Autodesk Fusion 360 part; units mm, degrees
(part 4 of 5)
  line L581 (-46.6267, 18.3537, 609.9137) -> (-48.3447, 10.2533, 610.9671) construction
  line L582 (-48.3447, 10.2533, 610.9671) -> (-50.0626, 2.1529, 612.0205) construction
  line L583 (-50.0626, 2.1529, 612.0205) -> (-49.7012, -6.3796, 613.0739) construction
  line L584 (-49.7012, -6.3796, 613.0739) -> (-47.3042, -14.3056, 614.1273) construction
  line L585 (-47.3042, -14.3056, 614.1273) -> (-44.9073, -22.2315, 615.1807) construction
  line L586 (-44.9073, -22.2315, 615.1807) -> (-40.48, -29.5343, 616.2341) construction
  line L587 (-40.48, -29.5343, 616.2341) -> (-34.5612, -35.325, 617.2875) construction
  line L588 (-34.5612, -35.325, 617.2875) -> (-28.6425, -41.1158, 618.3408) construction
  line L589 (-28.6425, -41.1158, 618.3408) -> (-21.2448, -45.3823, 619.3942) construction
  line L590 (-21.2448, -45.3823, 619.3942) -> (-13.2686, -47.6055, 620.4476) construction
  line L591 (-13.2686, -47.6055, 620.4476) -> (-5.2924, -49.8286, 621.5009) construction
  line L592 (-5.2924, -49.8286, 621.5009) -> (3.2455, -50.0036, 622.5543) construction
  line L593 (3.2455, -50.0036, 622.5543) -> (11.3061, -48.1093, 623.6076) construction
  line L594 (11.3061, -48.1093, 623.6076) -> (19.3665, -46.2151, 624.661) construction
  line L595 (19.3665, -46.2151, 624.661) -> (26.9327, -42.2555, 625.7143) construction
  line L596 (26.9327, -42.2555, 625.7143) -> (33.0837, -36.7125, 626.7677) construction
  line L597 (33.0837, -36.7125, 626.7677) -> (39.2345, -31.1696, 627.821) construction
  line L598 (39.2345, -31.1696, 627.821) -> (43.9574, -24.055, 628.8743) construction
  line L599 (43.9574, -24.055, 628.8743) -> (46.6773, -16.2346, 629.9277) construction
  line L600 (46.6773, -16.2346, 629.9277) -> (49.3973, -8.4143, 630.981) construction
  line L601 (49.3973, -8.4143, 630.981) -> (50.1087, 0.0954, 632.0343) construction
  line L602 (50.1087, 0.0954, 632.0343) -> (48.725, 8.2588, 633.0876) construction
  line L603 (48.725, 8.2588, 633.0876) -> (47.3414, 16.422, 634.1409) construction
  line L604 (47.3414, 16.422, 634.1409) -> (43.8656, 24.2219, 635.1942) construction
  line L605 (43.8656, 24.2219, 635.1942) -> (38.7207, 30.709, 636.2475) construction
  line L606 (38.7207, 30.709, 636.2475) -> (33.5759, 37.1961, 637.3008) construction
  line L607 (33.5759, 37.1961, 637.3008) -> (26.7728, 42.3569, 638.354) construction
  line L608 (26.7728, 42.3569, 638.354) -> (19.1393, 45.5634, 639.4073) construction
  line L609 (19.1393, 45.5634, 639.4073) -> (11.506, 48.7699, 640.4606) construction
  line L610 (11.506, 48.7699, 640.4606) -> (3.0583, 50.0153, 641.5139) construction
  line L611 (3.0583, 50.0153, 641.5139) -> (-5.1756, 49.1482, 642.5671) construction
  line L612 (-5.1756, 49.1482, 642.5671) -> (-13.4094, 48.2812, 643.6204) construction
  line L613 (-13.4094, 48.2812, 643.6204) -> (-21.4122, 45.3034, 644.6736) construction
  line L614 (-21.4122, 45.3034, 644.6736) -> (-28.2102, 40.5774, 645.7269) construction
  line L615 (-28.2102, 40.5774, 645.7269) -> (-35.008, 35.8514, 646.7801) construction
  line L616 (-35.008, 35.8514, 646.7801) -> (-40.5867, 29.3871, 647.8334) construction
  line L617 (-40.5867, 29.3871, 647.8334) -> (-44.2675, 21.971, 648.8866) construction
  line L618 (-44.2675, 21.971, 648.8866) -> (-47.9482, 14.5551, 649.9398) construction
  line L619 (-47.9482, 14.5551, 649.9398) -> (-49.7233, 6.203, 650.993) construction
  line L620 (-49.7233, 6.203, 650.993) -> (-49.3767, -2.0688, 652.0463) construction
  line L621 (-49.3767, -2.0688, 652.0463) -> (-49.0301, -10.3405, 653.0995) construction
  line L622 (-49.0301, -10.3405, 653.0995) -> (-46.5627, -18.5147, 654.1527) construction
  line L623 (-46.5627, -18.5147, 654.1527) -> (-42.2746, -25.5967, 655.2059) construction
  line L624 (-42.2746, -25.5967, 655.2059) -> (-37.9867, -32.6786, 656.2591) construction
  line L625 (-37.9867, -32.6786, 656.2591) -> (-31.8871, -38.6534, 657.3123) construction
  line L626 (-31.8871, -38.6534, 657.3123) -> (-24.7182, -42.7942, 658.3655) construction
  line L627 (-24.7182, -42.7942, 658.3655) -> (-17.5494, -46.935, 659.4186) construction
  line L628 (-17.5494, -46.935, 659.4186) -> (-9.3262, -49.2331, 660.4718) construction
  line L629 (-9.3262, -49.2331, 660.4718) -> (-1.0493, -49.4089, 661.525) construction
  line L630 (-1.0493, -49.4089, 661.525) -> (7.2275, -49.5846, 662.5782) construction
  line L631 (7.2275, -49.5846, 662.5782) -> (15.5406, -47.6378, 663.6313) construction
  line L632 (15.5406, -47.6378, 663.6313) -> (22.8787, -43.8053, 664.6845) construction
  line L633 (22.8787, -43.8053, 664.6845) -> (30.2167, -39.9728, 665.7376) construction
  line L634 (30.2167, -39.9728, 665.7376) -> (36.5642, -34.2626, 666.7908) construction
  line L635 (36.5642, -34.2626, 666.7908) -> (41.149, -27.3696, 667.8439) construction
  line L636 (41.149, -27.3696, 667.8439) -> (45.7337, -20.4766, 668.8971) construction
  line L637 (45.7337, -20.4766, 668.8971) -> (48.5461, -12.4153, 669.9502) construction
  line L638 (48.5461, -12.4153, 669.9502) -> (49.2441, -4.1664, 671.0033) construction
  line L639 (49.2441, -4.1664, 671.0033) -> (49.942, 4.0825, 672.0565) construction
  line L640 (49.942, 4.0825, 672.0565) -> (48.524, 12.5016, 673.1096) construction
  line L641 (48.524, 12.5016, 673.1096) -> (45.1626, 20.0668, 674.1627) construction
  line L642 (45.1626, 20.0668, 674.1627) -> (41.8013, 27.6318, 675.2158) construction
  line L643 (41.8013, 27.6318, 675.2158) -> (36.5037, 34.3271, 676.2689) construction
  line L644 (36.5037, 34.3271, 676.2689) -> (29.9143, 39.3379, 677.322) construction
  line L645 (29.9143, 39.3379, 677.322) -> (23.325, 44.3487, 678.3751) construction
  line L646 (23.325, 44.3487, 678.3751) -> (15.4578, 47.6647, 679.4282) construction
  line L647 (15.4578, 47.6647, 679.4282) -> (7.2698, 48.8824, 680.4813) construction
  line L648 (7.2698, 48.8824, 680.4813) -> (-0.9181, 50.1001, 681.5344) construction
  line L649 (-0.9181, 50.1001, 681.5344) -> (-9.4097, 49.2171, 682.5875) construction
  line L650 (-9.4097, 49.2171, 682.5875) -> (-17.1719, 46.3407, 683.6405) construction
  line L651 (-17.1719, 46.3407, 683.6405) -> (-24.934, 43.4644, 684.6936) construction
  line L652 (-24.934, 43.4644, 684.6936) -> (-31.9504, 38.6009, 685.7467) construction
  line L653 (-31.9504, 38.6009, 685.7467) -> (-37.3677, 32.3418, 686.7997) construction
  line L654 (-37.3677, 32.3418, 686.7997) -> (-42.7849, 26.0828, 687.8528) construction
  line L655 (-42.7849, 26.0828, 687.8528) -> (-46.5916, 18.4414, 688.9058) construction
  line L656 (-46.5916, 18.4414, 688.9058) -> (-48.3247, 10.3471, 689.9589) construction
  line L657 (-48.3247, 10.3471, 689.9589) -> (-50.0578, 2.2529, 691.0119) construction
  line L658 (-50.0578, 2.2529, 691.0119) -> (-49.7137, -6.2772, 692.065) construction
  line L659 (-49.7137, -6.2772, 692.065) -> (-47.3344, -14.2055, 693.118) construction
  line L660 (-47.3344, -14.2055, 693.118) -> (-44.955, -22.1337, 694.171) construction
  line L661 (-44.955, -22.1337, 694.171) -> (-40.5455, -29.4435, 695.224) construction
  line L662 (-40.5455, -29.4435, 695.224) -> (-34.642, -35.2458, 696.2771) construction
  line L663 (-34.642, -35.2458, 696.2771) -> (-28.7386, -41.0481, 697.3301) construction
  line L664 (-28.7386, -41.0481, 697.3301) -> (-21.3538, -45.3306, 698.3831) construction
  line L665 (-21.3538, -45.3306, 698.3831) -> (-13.3858, -47.5726, 699.4361) construction
  line L666 (-13.3858, -47.5726, 699.4361) -> (-5.4179, -49.8146, 700.4891) construction
  line L667 (-5.4179, -49.8146, 700.4891) -> (3.1165, -50.0114, 701.5421) construction
  line L668 (3.1165, -50.0114, 701.5421) -> (11.1792, -48.139, 702.5951) construction
  line L669 (11.1792, -48.139, 702.5951) -> (19.2419, -46.2666, 703.6481) construction
  line L670 (19.2419, -46.2666, 703.6481) -> (26.816, -42.3291, 704.701) construction
  line L671 (26.816, -42.3291, 704.701) -> (32.9804, -36.8053, 705.754) construction
  line L672 (32.9804, -36.8053, 705.754) -> (39.1447, -31.2816, 706.807) construction
  line L673 (39.1447, -31.2816, 706.807) -> (43.8864, -24.1832, 707.86) construction
  line L674 (43.8864, -24.1832, 707.86) -> (46.6288, -16.3736, 708.9129) construction
  line L675 (46.6288, -16.3736, 708.9129) -> (49.3711, -8.5641, 709.9659) construction
  line L676 (49.3711, -8.5641, 709.9659) -> (50.1083, -0.0597, 711.0188) construction
  line L677 (50.1083, -0.0597, 711.0188) -> (48.7508, 8.1052, 712.0718) construction
  line L678 (48.7508, 8.1052, 712.0718) -> (47.3269, 16.6698, 713.1763) construction
  line L679 (47.3269, 16.6698, 713.1763) -> (43.597, 24.8399, 714.2808) construction
  line L680 (43.597, 24.8399, 714.2808) -> (38.0584, 31.5261, 715.3853) construction
  line L681 (38.0584, 31.5261, 715.3853) -> (32.5415, 38.1861, 716.4855) construction
  line L682 (32.5415, 38.1861, 716.4855) -> (25.2442, 43.3574, 717.5857) construction
  line L683 (25.2442, 43.3574, 717.5857) -> (17.1322, 46.3554, 718.6858) construction
  line L684 (17.1322, 46.3554, 718.6858) -> (9.0519, 49.3418, 719.7817) construction
  line L685 (9.0519, 49.3418, 719.7817) -> (0.1833, 50.1649, 720.8776) construction
  line L686 (0.1833, 50.1649, 720.8776) -> (-8.3086, 48.7166, 721.9735) construction
  line L687 (-8.3086, 48.7166, 721.9735) -> (-16.7673, 47.2739, 723.0651) construction
  line L688 (-16.7673, 47.2739, 723.0651) -> (-24.8317, 43.5816, 724.1567) construction
  line L689 (-24.8317, 43.5816, 724.1567) -> (-31.4507, 38.1207, 725.2483) construction
  line L690 (-31.4507, 38.1207, 725.2483) -> (-38.0438, 32.6812, 726.3357) construction
  line L691 (-38.0438, 32.6812, 726.3357) -> (-43.187, 25.5004, 727.423) construction
  line L692 (-43.187, 25.5004, 727.423) -> (-46.215, 17.5074, 728.5104) construction
  line L693 (-46.215, 17.5074, 728.5104) -> (-49.2311, 9.5456, 729.5935) construction
  line L694 (-49.2311, 9.5456, 729.5935) -> (-50.1417, 0.7969, 730.6766) construction
  line L695 (-50.1417, 0.7969, 730.6766) -> (-48.8297, -7.6154, 731.7597) construction
  line L696 (-48.8297, -7.6154, 731.7597) -> (-47.5229, -15.9948, 732.8385) construction
  line L697 (-47.5229, -15.9948, 732.8385) -> (-44.0143, -24.0209, 733.9174) construction
  line L698 (-44.0143, -24.0209, 733.9174) -> (-38.751, -30.6707, 734.9963) construction
  line L699 (-38.751, -30.6707, 734.9963) -> (-33.5084, -37.2946, 736.0709) construction
  line L700 (-33.5084, -37.2946, 736.0709) -> (-26.5371, -42.538, 737.1456) construction
  line L701 (-26.5371, -42.538, 737.1456) -> (-18.7189, -45.7377, 738.2202) construction
  line L702 (-18.7189, -45.7377, 738.2202) -> (-10.9313, -48.9249, 739.2907) construction
  line L703 (-10.9313, -48.9249, 739.2907) -> (-2.3212, -50.0775, 740.3611) construction
  line L704 (-2.3212, -50.0775, 740.3611) -> (6.0305, -49.0507, 741.4316) construction
  line L705 (6.0305, -49.0507, 741.4316) -> (14.3495, -48.0279, 742.4979) construction
  line L706 (14.3495, -48.0279, 742.4979) -> (22.3937, -44.8454, 743.5641) construction
  line L707 (22.3937, -44.8454, 743.5641) -> (29.1608, -39.8997, 744.6304) construction
  line L708 (29.1608, -39.8997, 744.6304) -> (35.9014, -34.9733, 745.6925) construction
  line L709 (35.9014, -34.9733, 745.6925) -> (41.3602, -28.3085, 746.7546) construction
  line L710 (41.3602, -28.3085, 746.7546) -> (44.8623, -20.7295, 747.8167) construction
  line L711 (44.8623, -20.7295, 747.8167) -> (48.3506, -13.1802, 748.8747) construction
  line L712 (48.3506, -13.1802, 748.8747) -> (49.8902, -4.7401, 749.9326) construction
  line L713 (49.8902, -4.7401, 749.9326) -> (49.292, 3.5547, 750.9906) construction
  line L714 (49.292, 3.5547, 750.9906) -> (48.6939, 11.8482, 752.0484) construction
  line L715 (48.6939, 11.8482, 752.0484) -> (45.96, 19.9789, 753.1062) construction
  line L716 (45.96, 19.9789, 753.1062) -> (41.4257, 26.9489, 754.164) construction
  line L717 (41.4257, 26.9489, 754.164) -> (36.8917, 33.9186, 755.2218) construction
  line L718 (36.8917, 33.9186, 755.2218) -> (30.5672, 39.7129, 756.2795) construction
  line L719 (30.5672, 39.7129, 756.2795) -> (23.2282, 43.621, 757.3372) construction
  line L720 (23.2282, 43.621, 757.3372) -> (15.8895, 47.5288, 758.3949) construction
  line L721 (15.8895, 47.5288, 758.3949) -> (7.5521, 49.5422, 759.4526) construction
  line L722 (7.5521, 49.5422, 759.4526) -> (-0.7612, 49.4141, 760.5103) construction
  line L723 (-0.7612, 49.4141, 760.5103) -> (-9.0741, 49.2861, 761.568) construction
  line L724 (-9.0741, 49.2861, 761.568) -> (-17.3451, 47.0171, 762.6256) construction
  line L725 (-17.3451, 47.0171, 762.6256) -> (-24.5596, 42.8854, 763.6833) construction
  line L726 (-24.5596, 42.8854, 763.6833) -> (-31.7739, 38.754, 764.7409) construction
  line L727 (-31.7739, 38.754, 764.7409) -> (-37.9163, 32.7689, 765.7985) construction
  line L728 (-37.9163, 32.7689, 765.7985) -> (-42.2336, 25.6644, 766.856) construction
  line L729 (-42.2336, 25.6644, 766.856) -> (-46.5506, 18.5602, 767.9136) construction
  line L730 (-46.5506, 18.5602, 767.9136) -> (-49.0335, 10.3518, 768.9711) construction
  line L731 (-49.0335, 10.3518, 768.9711) -> (-49.3776, 2.0458, 770.0287) construction
  line L732 (-49.3776, 2.0458, 770.0287) -> (-49.7218, -6.2597, 771.0862) construction
  line L733 (-49.7218, -6.2597, 771.0862) -> (-47.9266, -14.645, 772.1436) construction
  line L734 (-47.9266, -14.645, 772.1436) -> (-44.2124, -22.0817, 773.2011) construction
  line L735 (-44.2124, -22.0817, 773.2011) -> (-40.4984, -29.518, 774.2586) construction
  line L736 (-40.4984, -29.518, 774.2586) -> (-34.8733, -35.99, 775.316) construction
  line L737 (-34.8733, -35.99, 775.316) -> (-28.0271, -40.704, 776.3734) construction
  line L738 (-28.0271, -40.704, 776.3734) -> (-21.1812, -45.4179, 777.4308) construction
  line L739 (-21.1812, -45.4179, 777.4308) -> (-13.1288, -48.3638, 778.4882) construction
  line L740 (-13.1288, -48.3638, 778.4882) -> (-4.8572, -49.1807, 779.5456) construction
  line L741 (-4.8572, -49.1807, 779.5456) -> (3.414, -49.9976, 780.6029) construction
  line L742 (3.414, -49.9976, 780.6029) -> (11.8867, -48.6839, 781.6603) construction
  line L743 (11.8867, -48.6839, 781.6603) -> (19.5222, -45.4007, 782.7176) construction
  line L744 (19.5222, -45.4007, 782.7176) -> (27.1573, -42.1176, 783.7749) construction
  line L745 (27.1573, -42.1176, 783.7749) -> (33.939, -36.8722, 784.8322) construction
  line L746 (33.939, -36.8722, 784.8322) -> (39.0358, -30.3075, 785.8895) construction
  line L747 (39.0358, -30.3075, 785.8895) -> (44.1324, -23.7431, 786.9467) construction
  line L748 (44.1324, -23.7431, 786.9467) -> (47.5335, -15.8735, 788.0039) construction
  line L749 (47.5335, -15.8735, 788.0039) -> (48.8222, -7.6634, 789.0612) construction
  line L750 (48.8222, -7.6634, 789.0612) -> (50.1109, 0.5463, 790.1183) construction
  line L751 (50.1109, 0.5463, 790.1183) -> (49.2846, 9.0791, 791.1755) construction
  line L752 (49.2846, 9.0791, 791.1755) -> (46.4446, 16.889, 792.2327) construction
  line L753 (46.4446, 16.889, 792.2327) -> (43.6047, 24.6985, 793.2898) construction
  line L754 (43.6047, 24.6985, 793.2898) -> (38.7575, 31.7687, 794.347) construction
  line L755 (38.7575, 31.7687, 794.347) -> (32.4969, 37.2329, 795.4041) construction
  line L756 (32.4969, 37.2329, 795.4041) -> (26.2365, 42.6969, 796.4612) construction
  line L757 (26.2365, 42.6969, 796.4612) -> (18.5763, 46.5436, 797.5183) construction
  line L758 (18.5763, 46.5436, 797.5183) -> (10.4549, 48.3015, 798.5754) construction
  line L759 (10.4549, 48.3015, 798.5754) -> (2.3339, 50.0593, 799.6324) construction
  line L760 (2.3339, 50.0593, 799.6324) -> (-6.2309, 49.7248, 800.6894) construction
  line L761 (-6.2309, 49.7248, 800.6894) -> (-14.1901, 47.339, 801.7465) construction
  line L762 (-14.1901, 47.339, 801.7465) -> (-22.1489, 44.9533, 802.8034) construction
  line L763 (-22.1489, 44.9533, 802.8034) -> (-29.4851, 40.5216, 803.8604) construction
  line L764 (-29.4851, 40.5216, 803.8604) -> (-35.3, 34.5868, 804.9174) construction
  line L765 (-35.3, 34.5868, 804.9174) -> (-41.1146, 28.6523, 805.9743) construction
  line L766 (-41.1146, 28.6523, 805.9743) -> (-45.3955, 21.2275, 807.0313) construction
  line L767 (-45.3955, 21.2275, 807.0313) -> (-47.6184, 13.2221, 808.0882) construction
  line L768 (-47.6184, 13.2221, 808.0882) -> (-49.8411, 5.2171, 809.1451) construction
  line L769 (-49.8411, 5.2171, 809.1451) -> (-50.0013, -3.3515, 810.202) construction
  line L770 (-50.0013, -3.3515, 810.202) -> (-48.0791, -11.434, 811.2589) construction
  line L771 (-48.0791, -11.434, 811.2589) -> (-46.157, -19.5161, 812.3157) construction
  line L772 (-46.157, -19.5161, 812.3157) -> (-42.157, -27.0949, 813.3725) construction
  line L773 (-42.157, -27.0949, 813.3725) -> (-36.569, -33.2422, 814.4294) construction
  line L774 (-36.569, -33.2422, 814.4294) -> (-30.9812, -39.3892, 815.4862) construction
  line L775 (-30.9812, -39.3892, 815.4862) -> (-23.8175, -44.0916, 816.543) construction
  line L776 (-23.8175, -44.0916, 816.543) -> (-15.9552, -46.7736, 817.5997) construction
  line L777 (-15.9552, -46.7736, 817.5997) -> (-8.0933, -49.4554, 818.6565) construction
  line L778 (-8.0933, -49.4554, 818.6565) -> (0.4504, -50.1112, 819.7132) construction
  line L779 (0.4504, -50.1112, 819.7132) -> (8.6296, -48.6607, 820.77) construction
  line L780 (8.6296, -48.6607, 820.77) -> (16.8083, -47.2103, 821.8267) construction
  line L781 (16.8083, -47.2103, 821.8267) -> (24.6051, -43.6568, 822.8833) construction
  line L782 (24.6051, -43.6568, 822.8833) -> (31.0653, -38.4355, 823.94) construction
  line L783 (31.0653, -38.4355, 823.94) -> (37.5251, -33.2143, 824.9967) construction
  line L784 (37.5251, -33.2143, 824.9967) -> (42.6346, -26.3366, 826.0533) construction
  line L785 (42.6346, -26.3366, 826.0533) -> (45.7682, -18.6443, 827.11) construction
  line L786 (45.7682, -18.6443, 827.11) -> (48.9016, -10.9525, 828.1666) construction
  line L787 (48.9016, -10.9525, 828.1666) -> (50.0525, -2.4625, 829.2232) construction
  line L788 (50.0525, -2.4625, 829.2232) -> (49.0801, 5.786, 830.2798) construction
  line L789 (49.0801, 5.786, 830.2798) -> (48.1078, 14.0341, 831.3363) construction
  line L790 (48.1078, 14.0341, 831.3363) -> (45.0143, 22.0233, 832.3928) construction
  line L791 (45.0143, 22.0233, 832.3928) -> (40.1785, 28.7755, 833.4494) construction
  line L792 (40.1785, 28.7755, 833.4494) -> (35.3428, 35.5273, 834.5059) construction
  line L793 (35.3428, 35.5273, 834.5059) -> (28.7753, 41.0279, 835.5624) construction
  line L794 (28.7753, 41.0279, 835.5624) -> (21.2797, 44.6039, 836.6189) construction
  line L795 (21.2797, 44.6039, 836.6189) -> (13.7845, 48.1798, 837.6754) construction
  line L796 (13.7845, 48.1798, 837.6754) -> (5.3773, 49.8235, 838.7318) construction
  line L797 (5.3773, 49.8235, 838.7318) -> (-2.9127, 49.3341, 839.7883) construction
  line L798 (-2.9127, 49.3341, 839.7883) -> (-11.2024, 48.8447, 840.8447) construction
  line L799 (-11.2024, 48.8447, 840.8447) -> (-19.3574, 46.2232, 841.9011) construction
  line L800 (-19.3574, 46.2232, 841.9011) -> (-26.3796, 41.7906, 842.9575) construction
  line L801 (-26.3796, 41.7906, 842.9575) -> (-33.4014, 37.3582, 844.0138) construction
  line L802 (-33.4014, 37.3582, 844.0138) -> (-39.2756, 31.1242, 845.0702) construction
  line L803 (-39.2756, 31.1242, 845.0702) -> (-43.2833, 23.8515, 846.1266) construction
  line L804 (-43.2833, 23.8515, 846.1266) -> (-47.2907, 16.5792, 847.1829) construction
  line L805 (-47.2907, 16.5792, 847.1829) -> (-49.4233, 8.2838, 848.2392) construction
  line L806 (-49.4233, 8.2838, 848.2392) -> (-49.42, -0.0196, 849.2955) construction
  line L807 (-49.42, -0.0196, 849.2955) -> (-49.4167, -8.3227, 850.3518) construction
  line L808 (-49.4167, -8.3227, 850.3518) -> (-47.2777, -16.616, 851.408) construction
  line L809 (-47.2777, -16.616, 851.408) -> (-43.2648, -23.8849, 852.4643) construction
  line L810 (-43.2648, -23.8849, 852.4643) -> (-39.2521, -31.1535, 853.5205) construction
  line L811 (-39.2521, -31.1535, 853.5205) -> (-33.3741, -37.3823, 854.5767) construction
  line L812 (-33.3741, -37.3823, 854.5767) -> (-26.3501, -41.8092, 855.633) construction
  line L813 (-26.3501, -41.8092, 855.633) -> (-19.3263, -46.2359, 856.6891) construction
  line L814 (-19.3263, -46.2359, 856.6891) -> (-11.1715, -48.8514, 857.7453) construction
  line L815 (-11.1715, -48.8514, 857.7453) -> (-2.8834, -49.3358, 858.8015) construction
  line L816 (-2.8834, -49.3358, 858.8015) -> (5.4044, -49.8202, 859.8576) construction
  line L817 (5.4044, -49.8202, 859.8576) -> (13.808, -48.1726, 860.9137) construction
  line L818 (13.808, -48.1726, 860.9137) -> (21.2994, -44.5945, 861.9699) construction
  line L819 (21.2994, -44.5945, 861.9699) -> (28.7904, -41.0167, 863.026) construction
  line L820 (28.7904, -41.0167, 863.026) -> (35.3533, -35.5161, 864.082) construction
  line L821 (35.3533, -35.5161, 864.082) -> (40.1854, -28.7657, 865.1381) construction
  line L822 (40.1854, -28.7657, 865.1381) -> (45.0173, -22.0157, 866.1942) construction
  line L823 (45.0173, -22.0157, 866.1942) -> (48.1082, -14.0302, 867.2502) construction
  line L824 (48.1082, -14.0302, 867.2502) -> (49.0801, -5.786, 868.3062) construction
  line L825 (49.0801, -5.786, 868.3062) -> (50.052, 2.4578, 869.3622) construction
  line L826 (50.052, 2.4578, 869.3622) -> (48.9029, 10.9427, 870.4182) construction
  line L827 (48.9029, 10.9427, 870.4182) -> (45.7735, 18.6311, 871.4742) construction
  line L828 (45.7735, 18.6311, 871.4742) -> (42.6443, 26.3192, 872.5302) construction
  line L829 (42.6443, 26.3192, 872.5302) -> (37.5414, 33.1945, 873.5861) construction
  line L830 (37.5414, 33.1945, 873.5861) -> (31.0891, 38.4162, 874.6421) construction
  line L831 (31.0891, 38.4162, 874.6421) -> (24.637, 43.6377, 875.698) construction
  line L832 (24.637, 43.6377, 875.698) -> (16.8492, 47.1946, 876.7539) construction
  line L833 (16.8492, 47.1946, 876.7539) -> (8.678, 48.6521, 877.8098) construction
  line L834 (8.678, 48.6521, 877.8098) -> (0.5071, 50.1095, 878.8656) construction
  line L835 (0.5071, 50.1095, 878.8656) -> (-8.0298, 49.4646, 879.9215) construction
  line L836 (-8.0298, 49.4646, 879.9215) -> (-15.889, 46.7961, 880.9774) construction
  line L837 (-15.889, 46.7961, 880.9774) -> (-23.7478, 44.1277, 882.0332) construction
  line L838 (-23.7478, 44.1277, 882.0332) -> (-30.9123, 39.4417, 883.089) construction
  line L839 (-30.9123, 39.4417, 883.089) -> (-36.5065, 33.3109, 884.1448) construction
  line L840 (-36.5065, 33.3109, 884.1448) -> (-42.1004, 27.1803, 885.2006) construction
  line L841 (-42.1004, 27.1803, 885.2006) -> (-46.1123, 19.6181, 886.2564) construction
  line L842 (-46.1123, 19.6181, 886.2564) -> (-48.0517, 11.5487, 887.3121) construction
  line L843 (-48.0517, 11.5487, 887.3121) -> (-49.991, 3.4797, 888.3678) construction
  line L844 (-49.991, 3.4797, 888.3678) -> (-49.8539, -5.0793, 889.4236) construction
  line L845 (-49.8539, -5.0793, 889.4236) -> (-47.6571, -13.0821, 890.4793) construction
  line L846 (-47.6571, -13.0821, 890.4793) -> (-45.4604, -21.0845, 891.535) construction
  line L847 (-45.4604, -21.0845, 891.535) -> (-41.2088, -28.5138, 892.5907) construction
  line L848 (-41.2088, -28.5138, 892.5907) -> (-35.4221, -34.4617, 893.6464) construction
  line L849 (-35.4221, -34.4617, 893.6464) -> (-29.6356, -40.4095, 894.702) construction
  line L850 (-29.6356, -40.4095, 894.702) -> (-22.3264, -44.8634, 895.7576) construction
  line L851 (-22.3264, -44.8634, 895.7576) -> (-14.3877, -47.2793, 896.8133) construction
  line L852 (-14.3877, -47.2793, 896.8133) -> (-6.4494, -49.695, 897.8689) construction
  line L853 (-6.4494, -49.695, 897.8689) -> (2.1015, -50.0677, 898.9245) construction
  line L854 (2.1015, -50.0677, 898.9245) -> (10.2199, -48.3517, 899.9801) construction
  line L855 (10.2199, -48.3517, 899.9801) -> (18.338, -46.6358, 901.0356) construction
  line L856 (18.338, -46.6358, 901.0356) -> (26.0065, -42.8351, 902.0912) construction
  line L857 (26.0065, -42.8351, 902.0912) -> (32.2882, -37.4141, 903.1467) construction
  line L858 (32.2882, -37.4141, 903.1467) -> (38.5696, -31.9932, 904.2023) construction
  line L859 (38.5696, -31.9932, 904.2023) -> (43.4511, -24.9636, 905.2578) construction
  line L860 (43.4511, -24.9636, 905.2578) -> (46.3361, -17.1843, 906.3133) construction
  line L861 (46.3361, -17.1843, 906.3133) -> (49.2211, -9.4052, 907.3687) construction
  line L862 (49.2211, -9.4052, 907.3687) -> (50.1036, -0.8929, 908.4242) construction
  line L863 (50.1036, -0.8929, 908.4242) -> (48.876, 7.3125, 909.4797) construction
  line L864 (48.876, 7.3125, 909.4797) -> (47.6484, 15.5176, 910.5351) construction
  line L865 (47.6484, 15.5176, 910.5351) -> (44.3134, 23.3986, 911.5905) construction
  line L866 (44.3134, 23.3986, 911.5905) -> (39.2784, 29.9925, 912.646) construction
  line L867 (39.2784, 29.9925, 912.646) -> (34.2435, 36.5861, 913.7014) construction
  line L868 (34.2435, 36.5861, 913.7014) -> (27.5195, 41.8788, 914.7567) construction
  line L869 (27.5195, 41.8788, 914.7567) -> (19.9278, 45.2241, 915.8121) construction
  line L870 (19.9278, 45.2241, 915.8121) -> (12.3363, 48.5692, 916.8675) construction
  line L871 (12.3363, 48.5692, 916.8675) -> (3.8933, 49.96, 917.9228) construction
  line L872 (3.8933, 49.96, 917.9228) -> (-4.37, 49.2264, 918.9782) construction
  line L873 (-4.37, 49.2264, 918.9782) -> (-12.633, 48.4929, 920.0335) construction
  line L874 (-12.633, 48.4929, 920.0335) -> (-20.6987, 45.6368, 921.0888) construction
  line L875 (-20.6987, 45.6368, 921.0888) -> (-27.582, 41.007, 922.1441) construction
  line L876 (-27.582, 41.007, 922.1441) -> (-34.465, 36.3774, 923.1993) construction
  line L877 (-34.465, 36.3774, 923.1993) -> (-40.151, 29.984, 924.2546) construction
  line L878 (-40.151, 29.984, 924.2546) -> (-43.9457, 22.6077, 925.3098) construction
  line L879 (-43.9457, 22.6077, 925.3098) -> (-47.7403, 15.2317, 926.3651) construction
  line L880 (-47.7403, 15.2317, 926.3651) -> (-49.6356, 6.8885, 927.4203) construction
  line L881 (-49.6356, 6.8885, 927.4203) -> (-49.4001, -1.4029, 928.4755) construction
  line L882 (-49.4001, -1.4029, 928.4755) -> (-49.1646, -9.6941, 929.5307) construction
  line L883 (-49.1646, -9.6941, 929.5307) -> (-46.7991, -17.9159, 930.5859) construction
  line L884 (-46.7991, -17.9159, 930.5859) -> (-42.5923, -25.0645, 931.641) construction
  line L885 (-42.5923, -25.0645, 931.641) -> (-38.3858, -32.2128, 932.6962) construction
  line L886 (-38.3858, -32.2128, 932.6962) -> (-32.347, -38.2727, 933.7513) construction
  line L887 (-32.347, -38.2727, 933.7513) -> (-25.2135, -42.5043, 934.8064) construction
  line L888 (-25.2135, -42.5043, 934.8064) -> (-18.0803, -46.7357, 935.8615) construction
  line L889 (-18.0803, -46.7357, 935.8615) -> (-9.8675, -49.13, 936.9166) construction
  line L890 (-9.8675, -49.13, 936.9166) -> (-1.5779, -49.3948, 937.9717) construction
  line L891 (-1.5779, -49.3948, 937.9717) -> (6.7114, -49.6596, 939.0268) construction
  line L892 (6.7114, -49.6596, 939.0268) -> (15.06, -47.7945, 940.0818) construction
  line L893 (15.06, -47.7945, 940.0818) -> (22.4485, -44.0273, 941.1369) construction
  line L894 (22.4485, -44.0273, 941.1369) -> (29.8367, -40.2602, 942.1919) construction
  line L895 (29.8367, -40.2602, 942.1919) -> (36.2494, -34.599, 943.2469) construction
  line L896 (36.2494, -34.599, 943.2469) -> (40.9036, -27.735, 944.302) construction
  line L897 (40.9036, -27.735, 944.302) -> (45.5577, -20.8711, 945.3569) construction
  line L898 (45.5577, -20.8711, 945.3569) -> (48.4436, -12.819, 946.4119) construction
  line L899 (48.4436, -12.819, 946.4119) -> (49.209, -4.5615, 947.4669) construction
  line L900 (49.209, -4.5615, 947.4669) -> (49.9744, 3.6957, 948.5218) construction
  line L901 (49.9744, 3.6957, 948.5218) -> (48.618, 12.1407, 949.5768) construction
  line L902 (48.618, 12.1407, 949.5768) -> (45.3051, 19.7428, 950.6317) construction
  line L903 (45.3051, 19.7428, 950.6317) -> (41.9925, 27.3447, 951.6866) construction
  line L904 (41.9925, 27.3447, 951.6866) -> (36.7306, 34.0875, 952.7415) construction
  line L905 (36.7306, 34.0875, 952.7415) -> (30.1618, 39.1485, 953.7964) construction
  line L906 (30.1618, 39.1485, 953.7964) -> (23.5933, 44.2092, 954.8512) construction
  line L907 (23.5933, 44.2092, 954.8512) -> (15.7318, 47.5774, 955.9061) construction
  line L908 (15.7318, 47.5774, 955.9061) -> (7.5368, 48.8419, 956.961) construction
  line L909 (7.5368, 48.8419, 956.961) -> (-0.6579, 50.1064, 958.0158) construction
  line L910 (-0.6579, 50.1064, 958.0158) -> (-9.1687, 49.2648, 959.0706) construction
  line L911 (-9.1687, 49.2648, 959.0706) -> (-16.9569, 46.4198, 960.1254) construction
  line L912 (-16.9569, 46.4198, 960.1254) -> (-24.7449, 43.5749, 961.1802) construction
  line L913 (-24.7449, 43.5749, 961.1802) -> (-31.794, 38.7327, 962.235) construction
  line L914 (-31.794, 38.7327, 962.235) -> (-37.244, 32.4842, 963.2897) construction
  line L915 (-37.244, 32.4842, 963.2897) -> (-42.6938, 26.2359, 964.3445) construction
  line L916 (-42.6938, 26.2359, 964.3445) -> (-46.533, 18.5945, 965.3992) construction
  line L917 (-46.533, 18.5945, 965.3992) -> (-48.2933, 10.4925, 966.454) construction
  line L918 (-48.2933, 10.4925, 966.454) -> (-50.0535, 2.3907, 967.5087) construction
  line L919 (-50.0535, 2.3907, 967.5087) -> (-49.7312, -6.1545, 968.5634) construction
  line L920 (-49.7312, -6.1545, 968.5634) -> (-47.3657, -14.1006, 969.6181) construction
  line L921 (-47.3657, -14.1006, 969.6181) -> (-45.0003, -22.0464, 970.6727) construction
  line L922 (-45.0003, -22.0464, 970.6727) -> (-40.5968, -29.3764, 971.7274) construction
  line L923 (-40.5968, -29.3764, 971.7274) -> (-34.6924, -35.1962, 972.7821) construction
  line L924 (-34.6924, -35.1962, 972.7821) -> (-28.7883, -41.0158, 973.8367) construction
  line L925 (-28.7883, -41.0158, 973.8367) -> (-21.3959, -45.3131, 974.8913) construction
  line L926 (-21.3959, -45.3131, 974.8913) -> (-13.4172, -47.5638, 975.9459) construction
  line L927 (-13.4172, -47.5638, 975.9459) -> (-5.4387, -49.8144, 977.0005) construction
  line L928 (-5.4387, -49.8144, 977.0005) -> (3.1093, -50.0139, 978.0551) construction
  line L929 (3.1093, -50.0139, 978.0551) -> (11.1841, -48.1379, 979.1097) construction
  line L930 (11.1841, -48.1379, 979.1097) -> (19.2586, -46.2619, 980.1643) construction
  line L931 (19.2586, -46.2619, 980.1643) -> (26.8428, -42.3145, 981.2188) construction
  line L932 (26.8428, -42.3145, 981.2188) -> (33.0117, -36.7772, 982.2734) construction
  line L933 (33.0117, -36.7772, 982.2734) -> (39.1804, -31.2402, 983.3279) construction
  line L934 (39.1804, -31.2402, 983.3279) -> (43.9208, -24.125, 984.3824) construction
  line L935 (43.9208, -24.125, 984.3824) -> (46.6547, -16.2996, 985.4369) construction
  line L936 (46.6547, -16.2996, 985.4369) -> (49.3885, -8.4744, 986.4914) construction
  line L937 (49.3885, -8.4744, 986.4914) -> (50.1103, 0.0444, 987.5458) construction
  line L938 (50.1103, 0.0444, 987.5458) -> (48.7319, 8.218, 988.6003) construction
  line L939 (48.7319, 8.218, 988.6003) -> (47.3536, 16.3912, 989.6548) construction
  line L940 (47.3536, 16.3912, 989.6548) -> (43.8783, 24.202, 990.7092) construction
  line L941 (43.8783, 24.202, 990.7092) -> (38.7297, 30.6977, 991.7636) construction
  line L942 (38.7297, 30.6977, 991.7636) -> (33.5813, 37.1932, 992.818) construction
  line L943 (33.5813, 37.1932, 992.818) -> (26.7706, 42.36, 993.8724) construction
  line L944 (26.7706, 42.36, 993.8724) -> (19.1283, 45.568, 994.9268) construction
  line L945 (19.1283, 45.568, 994.9268) -> (11.4862, 48.776, 995.9812) construction
  line L946 (11.4862, 48.776, 995.9812) -> (3.0286, 50.0186, 997.0356) construction
  line L947 (3.0286, 50.0186, 997.0356) -> (-5.2133, 49.1443, 998.0899) construction
  line L948 (-5.2133, 49.1443, 998.0899) -> (-13.4548, 48.27, 999.1443) construction
  line L949 (-13.4548, 48.27, 999.1443) -> (-21.4633, 45.2808, 1000.1986) construction
  line L950 (-21.4633, 45.2808, 1000.1986) -> (-28.2621, 40.5412, 1001.2529) construction
  line L951 (-28.2621, 40.5412, 1001.2529) -> (-35.0607, 35.8018, 1002.3072) construction
  line L952 (-35.0607, 35.8018, 1002.3072) -> (-40.6354, 29.3221, 1003.3615) construction
  line L953 (-40.6354, 29.3221, 1003.3615) -> (-44.3066, 21.892, 1004.4158) construction
  line L954 (-44.3066, 21.892, 1004.4158) -> (-47.9777, 14.4623, 1005.4701) construction
  line L955 (-47.9777, 14.4623, 1005.4701) -> (-49.7376, 6.098, 1006.5243) construction
  line L956 (-49.7376, 6.098, 1006.5243) -> (-49.3718, -2.1812, 1007.5786) construction
  line L957 (-49.3718, -2.1812, 1007.5786) -> (-49.0061, -10.4601, 1008.6328) construction
  line L958 (-49.0061, -10.4601, 1008.6328) -> (-46.5156, -18.6363, 1009.687) construction
  line L959 (-46.5156, -18.6363, 1009.687) -> (-42.2038, -25.7133, 1010.7412) construction
  line L960 (-42.2038, -25.7133, 1010.7412) -> (-37.8923, -32.7899, 1011.7954) construction
  line L961 (-37.8923, -32.7899, 1011.7954) -> (-31.7688, -38.7524, 1012.8496) construction
  line L962 (-31.7688, -38.7524, 1012.8496) -> (-24.5797, -42.8739, 1013.9038) construction
  line L963 (-24.5797, -42.8739, 1013.9038) -> (-17.3909, -46.9953, 1014.9579) construction
  line L964 (-17.3909, -46.9953, 1014.9579) -> (-9.1518, -49.2671, 1016.0121) construction
  line L965 (-9.1518, -49.2671, 1016.0121) -> (-0.8667, -49.4124, 1017.0662) construction
  line L966 (-0.8667, -49.4124, 1017.0662) -> (7.4181, -49.5577, 1018.1204) construction
  line L967 (7.4181, -49.5577, 1018.1204) -> (15.7316, -47.5764, 1019.1745) construction
  line L968 (15.7316, -47.5764, 1019.1745) -> (23.0603, -43.7099, 1020.2286) construction
  line L969 (23.0603, -43.7099, 1020.2286) -> (30.3888, -39.8436, 1021.2827) construction
  line L970 (30.3888, -39.8436, 1021.2827) -> (36.7172, -34.1004, 1022.3367) construction
  line L971 (36.7172, -34.1004, 1022.3367) -> (41.2743, -27.1803, 1023.3908) construction
  line L972 (41.2743, -27.1803, 1023.3908) -> (45.8312, -20.2604, 1024.4449) construction
  line L973 (45.8312, -20.2604, 1024.4449) -> (48.6074, -12.1782, 1025.4989) construction
  line L974 (48.6074, -12.1782, 1025.4989) -> (49.2644, -3.9188, 1026.553) construction
  line L975 (49.2644, -3.9188, 1026.553) -> (49.9214, 4.3404, 1027.607) construction
  line L976 (49.9214, 4.3404, 1027.607) -> (48.458, 12.7596, 1028.661) construction
  line L977 (48.458, 12.7596, 1028.661) -> (45.0525, 20.3127, 1029.715) construction
  line L978 (45.0525, 20.3127, 1029.715) -> (41.6472, 27.8655, 1030.769) construction
  line L979 (41.6472, 27.8655, 1030.769) -> (36.3072, 34.5365, 1031.8229) construction
  line L980 (36.3072, 34.5365, 1031.8229) -> (29.683, 39.5127, 1032.8769) construction
  line L981 (29.683, 39.5127, 1032.8769) -> (23.0591, 44.4888, 1033.9309) construction
  line L982 (23.0591, 44.4888, 1033.9309) -> (15.1652, 47.7597, 1034.9848) construction
  line L983 (15.1652, 47.7597, 1034.9848) -> (6.9631, 48.927, 1036.0387) construction
  line L984 (6.9631, 48.927, 1036.0387) -> (-1.2387, 50.0943, 1037.0926) construction
  line L985 (-1.2387, 50.0943, 1037.0926) -> (-9.7315, 49.1555, 1038.1466) construction
  line L986 (-9.7315, 49.1555, 1038.1466) -> (-17.4804, 46.2252, 1039.2005) construction
  line L987 (-17.4804, 46.2252, 1039.2005) -> (-25.2291, 43.295, 1040.2543) construction
  line L988 (-25.2291, 43.295, 1040.2543) -> (-32.2177, 38.3794, 1041.3082) construction
  line L989 (-32.2177, 38.3794, 1041.3082) -> (-37.5949, 32.0775, 1042.3621) construction
  line L990 (-37.5949, 32.0775, 1042.3621) -> (-42.9718, 25.7757, 1043.4159) construction
  line L991 (-42.9718, 25.7757, 1043.4159) -> (-46.726, 18.1008, 1044.4698) construction
  line L992 (-46.726, 18.1008, 1044.4698) -> (-48.4002, 9.9877, 1045.5236) construction
  line L993 (-48.4002, 9.9877, 1045.5236) -> (-50.0744, 1.875, 1046.5774) construction
  line L994 (-50.0744, 1.875, 1046.5774) -> (-49.665, -6.6588, 1047.6312) construction
  line L995 (-49.665, -6.6588, 1047.6312) -> (-47.2221, -14.5741, 1048.685) construction
  line L996 (-47.2221, -14.5741, 1048.685) -> (-44.7793, -22.4892, 1049.7388) construction
  line L997 (-44.7793, -22.4892, 1049.7388) -> (-40.3082, -29.7691, 1050.7926) construction
  line L998 (-40.3082, -29.7691, 1050.7926) -> (-34.3534, -35.5272, 1051.8463) construction
  line L999 (-34.3534, -35.5272, 1051.8463) -> (-28.3987, -41.2851, 1052.9001) construction
  line L1000 (-28.3987, -41.2851, 1052.9001) -> (-20.973, -45.5091, 1053.9538) construction
  line L1001 (-20.973, -45.5091, 1053.9538) -> (-12.9807, -47.6848, 1055.0076) construction
  line L1002 (-12.9807, -47.6848, 1055.0076) -> (-4.9886, -49.8604, 1056.0613) construction
  line L1003 (-4.9886, -49.8604, 1056.0613) -> (3.5533, -49.9832, 1057.115) construction
  line L1004 (3.5533, -49.9832, 1057.115) -> (11.6047, -48.0382, 1058.1687) construction
  line L1005 (11.6047, -48.0382, 1058.1687) -> (19.6557, -46.0933, 1059.2224) construction
  line L1006 (19.6557, -46.0933, 1059.2224) -> (27.1994, -42.0848, 1060.276) construction
  line L1007 (27.1994, -42.0848, 1060.276) -> (33.3169, -36.501, 1061.3297) construction
  line L1008 (33.3169, -36.501, 1061.3297) -> (39.4342, -30.9174, 1062.3834) construction
  line L1009 (39.4342, -30.9174, 1062.3834) -> (44.1125, -23.7702, 1063.437) construction
  line L1010 (44.1125, -23.7702, 1063.437) -> (46.7822, -15.9298, 1064.4907) construction
  line L1011 (46.7822, -15.9298, 1064.4907) -> (49.4519, -8.0897, 1065.5443) construction
  line L1012 (49.4519, -8.0897, 1065.5443) -> (50.1074, 0.427, 1066.5979) construction
  line L1013 (50.1074, 0.427, 1066.5979) -> (48.6689, 8.5833, 1067.6515) construction
  line L1014 (48.6689, 8.5833, 1067.6515) -> (47.2305, 16.7394, 1068.7051) construction
  line L1015 (47.2305, 16.7394, 1068.7051) -> (43.7013, 24.5178, 1069.7586) construction
  line L1016 (43.7013, 24.5178, 1069.7586) -> (38.511, 30.9716, 1070.8122) construction
  line L1017 (38.511, 30.9716, 1070.8122) -> (33.3208, 37.4252, 1071.8658) construction
  line L1018 (33.3208, 37.4252, 1071.8658) -> (26.4807, 42.5405, 1072.9193) construction
  line L1019 (26.4807, 42.5405, 1072.9193) -> (18.8232, 45.6949, 1073.9729) construction
  line L1020 (18.8232, 45.6949, 1073.9729) -> (11.166, 48.8491, 1075.0264) construction
  line L1021 (11.166, 48.8491, 1075.0264) -> (2.7078, 50.0359, 1076.0799) construction
  line L1022 (2.7078, 50.0359, 1076.0799) -> (-5.5218, 49.1105, 1077.1334) construction
  line L1023 (-5.5218, 49.1105, 1077.1334) -> (-13.7511, 48.1853, 1078.1869) construction
  line L1024 (-13.7511, 48.1853, 1078.1869) -> (-21.7345, 45.1501, 1079.2404) construction
  line L1025 (-21.7345, 45.1501, 1079.2404) -> (-28.4999, 40.3744, 1080.2939) construction
  line L1026 (-28.4999, 40.3744, 1080.2939) -> (-35.2651, 35.5989, 1081.3473) construction
  line L1027 (-35.2651, 35.5989, 1081.3473) -> (-40.7983, 29.0931, 1082.4008) construction
  line L1028 (-40.7983, 29.0931, 1082.4008) -> (-44.4259, 21.649, 1083.4542) construction
  line L1029 (-44.4259, 21.649, 1083.4542) -> (-48.0533, 14.2051, 1084.5077) construction
  line L1030 (-48.0533, 14.2051, 1084.5077) -> (-49.7676, 5.8386, 1085.5611) construction
  line L1031 (-49.7676, 5.8386, 1085.5611) -> (-49.3601, -2.432, 1086.6145) construction
  line L1032 (-49.3601, -2.432, 1086.6145) -> (-48.9526, -10.7024, 1087.6679) construction
  line L1033 (-48.9526, -10.7024, 1087.6679) -> (-46.4243, -18.8597, 1088.7213) construction
  line L1034 (-46.4243, -18.8597, 1088.7213) -> (-42.0829, -25.9108, 1089.7747) construction
  line L1035 (-42.0829, -25.9108, 1089.7747) -> (-37.7416, -32.9616, 1090.8281) construction
  line L1036 (-37.7416, -32.9616, 1090.8281) -> (-31.5965, -38.8917, 1091.8814) construction
  line L1037 (-31.5965, -38.8917, 1091.8814) -> (-24.3954, -42.9791, 1092.9348) construction
  line L1038 (-24.3954, -42.9791, 1092.9348) -> (-17.1946, -47.0664, 1093.9881) construction
  line L1039 (-17.1946, -47.0664, 1093.9881) -> (-8.953, -49.3025, 1095.0414) construction
  line L1040 (-8.953, -49.3025, 1095.0414) -> (-0.6738, -49.4154, 1096.0948) construction
  line L1041 (-0.6738, -49.4154, 1096.0948) -> (7.6052, -49.5283, 1097.1481) construction
  line L1042 (7.6052, -49.5283, 1097.1481) -> (15.9044, -47.5178, 1098.2014) construction
  line L1043 (15.9044, -47.5178, 1098.2014) -> (23.2138, -43.6286, 1099.2547) construction
  line L1044 (23.2138, -43.6286, 1099.2547) -> (30.5231, -39.7395, 1100.308) construction
  line L1045 (30.5231, -39.7395, 1100.308) -> (36.8273, -33.98, 1101.3612) construction
  line L1046 (36.8273, -33.98, 1101.3612) -> (41.3592, -27.0509, 1102.4145) construction
  line L1047 (41.3592, -27.0509, 1102.4145) -> (45.891, -20.1221, 1103.4677) construction
  line L1048 (45.891, -20.1221, 1103.4677) -> (48.6412, -12.0383, 1104.521) construction
  line L1049 (48.6412, -12.0383, 1104.521) -> (49.275, -3.7833, 1105.5742) construction
  line L1050 (49.275, -3.7833, 1105.5742) -> (49.9088, 4.4714, 1106.6274) construction
  line L1051 (49.9088, 4.4714, 1106.6274) -> (48.425, 12.88, 1107.6807) construction
  line L1052 (48.425, 12.88, 1107.6807) -> (45.0043, 20.4193, 1108.7339) construction
  line L1053 (45.0043, 20.4193, 1108.7339) -> (41.5837, 27.9584, 1109.7871) construction
  line L1054 (41.5837, 27.9584, 1109.7871) -> (36.2333, 34.6124, 1110.8402) construction
  line L1055 (36.2333, 34.6124, 1110.8402) -> (29.6043, 39.5717, 1111.8934) construction
  line L1056 (29.6043, 39.5717, 1111.8934) -> (22.9755, 44.5309, 1112.9466) construction
  line L1057 (22.9755, 44.5309, 1112.9466) -> (15.0819, 47.785, 1113.9997) construction
  line L1058 (15.0819, 47.785, 1113.9997) -> (6.884, 48.9382, 1115.0529) construction
  line L1059 (6.884, 48.9382, 1115.0529) -> (-1.3136, 50.0913, 1116.106) construction
  line L1060 (-1.3136, 50.0913, 1116.106) -> (-9.7983, 49.1412, 1117.1591) construction
  line L1061 (-9.7983, 49.1412, 1117.1591) -> (-17.5379, 46.2034, 1118.2123) construction
  line L1062 (-17.5379, 46.2034, 1118.2123) -> (-25.2772, 43.2657, 1119.2654) construction
  line L1063 (-25.2772, 43.2657, 1119.2654) -> (-32.2552, 38.3467, 1120.3185) construction
  line L1064 (-32.2552, 38.3467, 1120.3185) -> (-37.6228, 32.0446, 1121.3716) construction
  line L1065 (-37.6228, 32.0446, 1121.3716) -> (-42.9904, 25.7428, 1122.4246) construction
  line L1066 (-42.9904, 25.7428, 1122.4246) -> (-46.7364, 18.0712, 1123.4777) construction
  line L1067 (-46.7364, 18.0712, 1123.4777) -> (-48.4053, 9.9633, 1124.5308) construction
  line L1068 (-48.4053, 9.9633, 1124.5308) -> (-50.0741, 1.8556, 1125.5838) construction
  line L1069 (-50.0741, 1.8556, 1125.5838) -> (-49.6623, -6.6715, 1126.6369) construction
  line L1070 (-49.6623, -6.6715, 1126.6369) -> (-47.2201, -14.5807, 1127.6899) construction
  line L1071 (-47.2201, -14.5807, 1127.6899) -> (-44.7779, -22.4897, 1128.7429) construction
  line L1072 (-44.7779, -22.4897, 1128.7429) -> (-40.3105, -29.7643, 1129.7959) construction
  line L1073 (-40.3105, -29.7643, 1129.7959) -> (-34.3613, -35.5195, 1130.8489) construction
  line L1074 (-34.3613, -35.5195, 1130.8489) -> (-28.4122, -41.2746, 1131.9019) construction
  line L1075 (-28.4122, -41.2746, 1131.9019) -> (-20.9938, -45.4984, 1132.9549) construction
  line L1076 (-20.9938, -45.4984, 1132.9549) -> (-13.0085, -47.6772, 1134.0079) construction
  line L1077 (-13.0085, -47.6772, 1134.0079) -> (-5.0233, -49.8559, 1135.0609) construction
  line L1078 (-5.0233, -49.8559, 1135.0609) -> (3.512, -49.9851, 1136.1138) construction
  line L1079 (3.512, -49.9851, 1136.1138) -> (11.5594, -48.0491, 1137.1668) construction
  line L1080 (11.5594, -48.0491, 1137.1668) -> (19.9816, -46.0229, 1138.2688) construction
  line L1081 (19.9816, -46.0229, 1138.2688) -> (27.8484, -41.7353, 1139.3707) construction
  line L1082 (27.8484, -41.7353, 1139.3707) -> (34.1157, -35.7555, 1140.4727) construction
  line L1083 (34.1157, -35.7555, 1140.4727) -> (40.334, -29.8223, 1141.5661) construction
  line L1084 (40.334, -29.8223, 1141.5661) -> (44.9628, -22.2385, 1142.6595) construction
  line L1085 (44.9628, -22.2385, 1142.6595) -> (47.3968, -13.9956, 1143.7529) construction
  line L1086 (47.3968, -13.9956, 1143.7529) -> (49.8118, -5.8171, 1144.8377) construction
  line L1087 (49.8118, -5.8171, 1144.8377) -> (50.0611, 2.9904, 1145.9225) construction
  line L1088 (50.0611, 2.9904, 1145.9225) -> (48.1126, 11.2924, 1147.0074) construction
  line L1089 (48.1126, 11.2924, 1147.0074) -> (46.1792, 19.5295, 1148.0837) construction
  line L1090 (46.1792, 19.5295, 1148.0837) -> (42.0875, 27.2501, 1149.1601) construction
  line L1091 (42.0875, 27.2501, 1149.1601) -> (36.3565, 33.4745, 1150.2364) construction
  line L1092 (36.3565, 33.4745, 1150.2364) -> (30.6702, 39.6503, 1151.3044) construction
  line L1093 (30.6702, 39.6503, 1151.3044) -> (23.3835, 44.3399, 1152.3723) construction
  line L1094 (23.3835, 44.3399, 1152.3723) -> (15.407, 46.957, 1153.4403) construction
  line L1095 (15.407, 46.957, 1153.4403) -> (7.4928, 49.5537, 1154.4999) construction
  line L1096 (7.4928, 49.5537, 1154.4999) -> (-1.083, 50.1053, 1155.5595) construction
  line L1097 (-1.083, 50.1053, 1155.5595) -> (-9.2646, 48.5438, 1156.6191) construction
  line L1098 (-9.2646, 48.5438, 1156.6191) -> (-17.432, 46.9851, 1157.6769) construction
  line L1099 (-17.432, 46.9851, 1157.6769) -> (-25.1892, 43.3241, 1158.7346) construction
  line L1100 (-25.1892, 43.3241, 1158.7346) -> (-31.5843, 38.0101, 1159.7924) construction
  line L1101 (-31.5843, 38.0101, 1159.7924) -> (-37.9789, 32.6966, 1160.8501) construction
  line L1102 (-37.9789, 32.6966, 1160.8501) -> (-42.9979, 25.7417, 1161.9077) construction
  line L1103 (-42.9979, 25.7417, 1161.9077) -> (-46.0259, 17.9987, 1162.9654) construction
  line L1104 (-46.0259, 17.9987, 1162.9654) -> (-49.0536, 10.2564, 1164.023) construction
  line L1105 (-49.0536, 10.2564, 1164.023) -> (-50.084, 1.7427, 1165.0805) construction
  line L1106 (-50.084, 1.7427, 1165.0805) -> (-48.9909, -6.4984, 1166.1381) construction
  line L1107 (-48.9909, -6.4984, 1166.1381) -> (-47.8979, -14.7386, 1167.1955) construction
  line L1108 (-47.8979, -14.7386, 1167.1955) -> (-44.684, -22.6886, 1168.253) construction
  line L1109 (-44.684, -22.6886, 1168.253) -> (-39.7435, -29.3734, 1169.3105) construction
  line L1110 (-39.7435, -29.3734, 1169.3105) -> (-34.8034, -36.0575, 1170.3678) construction
  line L1111 (-34.8034, -36.0575, 1170.3678) -> (-28.1474, -41.4625, 1171.4252) construction
  line L1112 (-28.1474, -41.4625, 1171.4252) -> (-20.5917, -44.9257, 1172.4825) construction
  line L1113 (-20.5917, -44.9257, 1172.4825) -> (-13.0367, -48.3885, 1173.5398) construction
  line L1114 (-13.0367, -48.3885, 1173.5398) -> (-4.5982, -49.9025, 1174.597) construction
  line L1115 (-4.5982, -49.9025, 1174.597) -> (3.6894, -49.2821, 1175.6543) construction
  line L1116 (3.6894, -49.2821, 1175.6543) -> (11.9762, -48.6617, 1176.7114) construction
  line L1117 (11.9762, -48.6617, 1176.7114) -> (20.0945, -45.9086, 1177.7686) construction
  line L1118 (20.0945, -45.9086, 1177.7686) -> (27.0493, -41.3603, 1178.8257) construction
  line L1119 (27.0493, -41.3603, 1178.8257) -> (34.0034, -36.8124, 1179.8828) construction
  line L1120 (34.0034, -36.8124, 1179.8828) -> (39.7794, -30.4792, 1180.9398) construction
  line L1121 (39.7794, -30.4792, 1180.9398) -> (43.6695, -23.1368, 1181.9969) construction
  line L1122 (43.6695, -23.1368, 1181.9969) -> (47.5592, -15.7952, 1183.0539) construction
  line L1123 (47.5592, -15.7952, 1183.0539) -> (49.5551, -7.4602, 1184.1108) construction
  line L1124 (49.5551, -7.4602, 1184.1108) -> (49.4127, 0.8471, 1185.1678) construction
  line L1125 (49.4127, 0.8471, 1185.1678) -> (49.2703, 9.1535, 1186.2246) construction
  line L1126 (49.2703, 9.1535, 1186.2246) -> (46.9903, 17.4145, 1187.2815) construction
  line L1127 (46.9903, 17.4145, 1187.2815) -> (42.8519, 24.618, 1188.3383) construction
  line L1128 (42.8519, 24.618, 1188.3383) -> (38.7139, 31.8209, 1189.3951) construction
  line L1129 (38.7139, 31.8209, 1189.3951) -> (32.7268, 37.9513, 1190.4518) construction
  line L1130 (32.7268, 37.9513, 1190.4518) -> (25.6236, 42.2583, 1191.5086) construction
  line L1131 (25.6236, 42.2583, 1191.5086) -> (18.5212, 46.5649, 1192.5653) construction
  line L1132 (18.5212, 46.5649, 1192.5653) -> (10.3181, 49.0394, 1193.6219) construction
  line L1133 (10.3181, 49.0394, 1193.6219) -> (2.0189, 49.3787, 1194.6786) construction
  line L1134 (2.0189, 49.3787, 1194.6786) -> (-6.2796, 49.718, 1195.7352) construction
  line L1135 (-6.2796, 49.718, 1195.7352) -> (-14.6565, 47.9218, 1196.7917) construction
  line L1136 (-14.6565, 47.9218, 1196.7917) -> (-22.0863, 44.2101, 1197.8483) construction
  line L1137 (-22.0863, 44.2101, 1197.8483) -> (-29.5155, 40.4986, 1198.9048) construction
  line L1138 (-29.5155, 40.4986, 1198.9048) -> (-35.9819, 34.8799, 1199.9612) construction
  line L1139 (-35.9819, 34.8799, 1199.9612) -> (-40.6941, 28.0415, 1201.0177) construction
  line L1140 (-40.6941, 28.0415, 1201.0177) -> (-45.4058, 21.2038, 1202.0741) construction
  line L1141 (-45.4058, 21.2038, 1202.0741) -> (-48.3536, 13.1613, 1203.1305) construction
  line L1142 (-48.3536, 13.1613, 1203.1305) -> (-49.1767, 4.8983, 1204.1868) construction
  line L1143 (-49.1767, 4.8983, 1204.1868) -> (-49.9996, -3.364, 1205.2431) construction
  line L1144 (-49.9996, -3.364, 1205.2431) -> (-48.6965, -11.8293, 1206.2994) construction
  line L1145 (-48.6965, -11.8293, 1206.2994) -> (-45.4267, -19.4615, 1207.3557) construction
  line L1146 (-45.4267, -19.4615, 1207.3557) -> (-42.1572, -27.0931, 1208.4119) construction
  line L1147 (-42.1572, -27.0931, 1208.4119) -> (-36.9284, -33.8757, 1209.4681) construction
  line L1148 (-36.9284, -33.8757, 1209.4681) -> (-30.3799, -38.9795, 1210.5243) construction